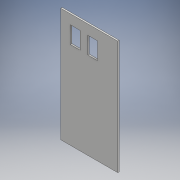
# Autodesk Inventor part: support_arriere
Saved by Autodesk Inventor 2017 (Build 210142000, 142)
## iProperties
Created: 2017-04-21
Part Number: support_arriere
Material: Generic
Document SubType Name: Modeling
Designer: franc
Density: 1 g/cm^3
Appearance: Default
Author: franc
Autodesk Inventor part; units mm, degrees
ref_plane "YZ Plane" through (0, 0, 0) normal (1, 0, 0) x (0, 1, 0)
ref_plane "XZ Plane" through (0, 0, 0) normal (0, 1, 0) x (-1, 0, 0)
ref_plane "XY Plane" through (0, 0, 0) normal (0, 0, 1) x (1, 0, 0)
sketch "Sketch1" plane through (0, 0, 0) normal (0, 1, 0) x (-1, 0, 0)
  line L0 (3.7718, 7.6653) -> (-146.2282, 7.6653)
  line L1 (-146.2282, 7.6653) -> (-146.2282, -292.3347)
  line L2 (-146.2282, -292.3347) -> (3.7718, -292.3347)
  line L3 (3.7718, -292.3347) -> (3.7718, 7.6653)
  line L4 (-21.2282, -17.3347) -> (-47.2282, -17.3347)
  line L5 (-47.2282, -17.3347) -> (-47.2282, -62.3347)
  line L6 (-47.2282, -62.3347) -> (-21.2282, -62.3347)
  line L7 (-21.2282, -62.3347) -> (-21.2282, -17.3347)
  line L8 (-67.2282, -18.3347) -> (-93.2282, -18.3347)
  line L9 (-93.2282, -18.3347) -> (-93.2282, -63.3347)
  line L10 (-93.2282, -63.3347) -> (-67.2282, -63.3347)
  line L11 (-67.2282, -63.3347) -> (-67.2282, -18.3347)
  point P0 (0, 0)
  dimension "d0" = 300
  dimension "d1" = 150
  dimension "d4" = 45
  dimension "d5" = 26
  dimension "d6" = 25
  dimension "d7" = 25
  dimension "d8" = 45
  dimension "d9" = 26
  dimension "d10" = 26
  dimension "d11" = 20
  constraints: 24 end point, 6 parallel, 3 horizontal, 3 perpendicular
  measures "d0" distance of L2.end L0.start
  measures "d1" distance of L0.start L0.end
  measures "d4" distance of L6.end L4.start
  measures "d5" distance of L5.end L6.end
  measures "d6" distance between parallel lines of L0 L4
  measures "d7" distance between parallel lines of L3 L7
  measures "d8" distance of L10.end L8.start
  measures "d9" distance of L9.end L10.end
  measures "d10" distance between parallel lines of L0 L8
  measures "d11" distance between parallel lines of L11 L5
extrude "Extrusion1" add sketch "Sketch1" along normal blind 4
body "Solid1"
